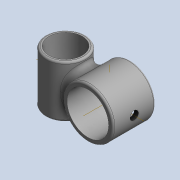
# Autodesk Inventor part: 45-76
Saved by Autodesk Inventor 2021 (Build 250183000, 183)
## iProperties
Created: 2020-04-23
Part Number: 45-76
Material: Generic
Document SubType Name: Modeling
Designer: Hannah
Density: 7.97385 g/cm^3
Appearance: Default
Mass: 450 g
Surface Area: 269.127 cm^2
Volume: 56.4345 cm^3
Author: Hannah
Autodesk Inventor part; units mm, degrees
ref_plane "XZ Plane" through (0, 0, 0) normal (0, 1, 0) x (-1, 0, 0)
ref_plane "XY Plane" through (0, 0, 0) normal (0, 0, 1) x (1, 0, 0)
sketch "Sketch1" plane through (0, 0, 0) normal (0, 0, 1) x (1, 0, 0)
  circle A0 centre (0, 0) radius 22
  circle A1 centre (0, 0) radius 26.5
  dimension "d1" = 53
  dimension "d2" = 44
  constraints: 2 centre point, 2 coincident
  measures "d1" diameter of A1
  measures "d2" diameter of A0
extrude "Extrusion1" add sketch "Sketch1" along normal mid plane 45 contours A0 | A1
sketch "Sketch2" plane through (0, 0, 0) normal (0, 1, 0) x (-1, 0, 0)
  circle A0 centre (46, 0) radius 17.5
  circle A1 centre (46, 0) radius 21
  line L0 (80.4, 0) -> (-13.4, 0) projected
  line L1 (0, -29.4) -> (0, 29.4) projected
  point P0 (0, 0)
  dimension "d5" = 35
  dimension "d6" = 42
  dimension "d13" = 46
  constraints: 2 centre point, 1 coincident, 1 point on line
  measures "d5" diameter of A0
  measures "d6" diameter of A1
  measures "d13" distance from line of L1 A0.centre
extrude "Extrusion2" add sketch "Sketch2" along normal mid plane 55
fillet "Fillet1" radius 5 4 edges at (-25.7953, 6.0707, 5.7244) (-25.7953, 6.0708, -5.7244) (-25.7953, -6.0708, -5.7244) (-25.7953, -6.0707, 5.7245)
extrude "Extrusion3" cut sketch "Sketch2" along normal through all both and the other way through all contours L0 A0 | A0 L0
extrude "Extrusion4" cut sketch "Sketch1" along normal through all both and the other way through all contours A0
hole "Hole1" at (0, 0, 0) direction (1, 0, 0) diameter 8.917 end through all thread size "M10x1" class "6H" standard "ISO Metric profile"
ref_plane "Work Plane1" through (-46, 0, 0) normal (1, 0, 0) x (0, 1, 0)
hole "Hole2" at (-46, 0, 0) direction (-1, 0, 0) diameter 8.917 end through all thread size "M10x1" class "6H" standard "ISO Metric profile"
fillet "Fillet2" radius 2 4 edges at (-25, 27.5, 0) (-25, -27.5, 0) (-26.5, 0, 22.5) (-26.5, 0, -22.5)
body "Solid1"
